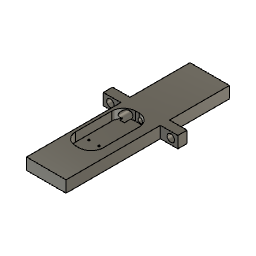
TRAY 3x1.5 v01.1 v3 (Autodesk Fusion 360 design; units mm, degrees)
Autodesk Fusion 360 part; units mm, degrees
sketch "Sketch1" plane through (0, 0, 0) normal (0, 0, 1) x (1, 0, 0)
  line L0 (0, 0) -> (43, 0)
  line L1 (43, 0) -> (43, 177.8)
  line L2 (43, 177.8) -> (0, 177.8)
  line L3 (0, 177.8) -> (0, 0)
  line L4 (0, 112.616) -> (-19.05, 112.616)
  line L5 (-19.05, 112.616) -> (-19.05, 102.616)
  line L6 (-19.05, 102.616) -> (0, 102.616)
  line L7 (0, 102.616) -> (0, 112.616)
  line L8 (43, 112.616) -> (62.05, 112.616)
  line L9 (62.05, 112.616) -> (62.05, 102.616)
  line L10 (62.05, 102.616) -> (43, 102.616)
  line L11 (43, 102.616) -> (43, 112.616)
  dimension "d1" = 177.8
  dimension "d2" = 43
  dimension "d5" = 75.184
  dimension "d6" = 75.184
  dimension "d7" = 10
  dimension "d8" = 10
  dimension "d9" = 19.05
  dimension "d10" = 19.05
  constraint horizontal L0
  constraint vertical L1
  constraint horizontal L2
  constraint vertical L3
  constraint coincident L0.start L3.end
  constraint horizontal L4
  constraint vertical L5
  constraint horizontal L6
  constraint vertical L7
  constraint coincident L3 L4.start
  constraint horizontal L8
  constraint vertical L9
  constraint horizontal L10
  constraint vertical L11
  constraint coincident L1 L8.start
  measures "d1" distance of L0.start L2.end
  measures "d2" distance of L1.end L2.end
  measures "d5" distance of L2.end L6
  measures "d6" distance of L2 L10
  measures "d7" distance of L4.end L5.end
  measures "d8" distance of L8.end L9.end
  measures "d9" distance of L4.start L4.end
  measures "d10" distance of L8.start L8.end
extrude "Extrude1" add sketch "Sketch1" along normal blind 12.6
sketch "Sketch2" plane through (0, 0, 12.6) normal (0, 0, 1) x (-1, 0, 0)
  line L0 (-43, -112.616) -> (-43, -177.8)
  line L1 (-43, -177.8) -> (0, -177.8)
  line L2 (0, -177.8) -> (0, -112.616)
  line L3 (0, -112.616) -> (19.05, -112.616)
  line L4 (19.05, -112.616) -> (19.05, -102.616)
  line L5 (19.05, -102.616) -> (0, -102.616)
  line L6 (0, -102.616) -> (0, 0)
  line L7 (0, 0) -> (-43, 0)
  line L8 (-43, 0) -> (-43, -102.616)
  line L9 (-43, -102.616) -> (-62.05, -102.616)
  line L10 (-62.05, -102.616) -> (-62.05, -112.616)
  line L11 (-62.05, -112.616) -> (-43, -112.616)
  line L12 (-3, -102.616) -> (-33, -102.616)
  line L13 (-33, -102.616) -> (-33, -37.316)
  line L14 (-33, -37.316) -> (-3, -37.316)
  line L15 (-3, -37.316) -> (-3, -102.616)
  dimension "d11" = 3
  dimension "d20" = 10
  dimension "d66" = 30
  dimension "d68" = 65.3
  constraint horizontal L12
  constraint vertical L13
  constraint horizontal L14
  constraint vertical L15
  measures "d11" distance of L6 L15
  measures "d20" distance of L3 L12
  measures "d66" distance of L12.start L12.end
  measures "d68" distance of L12.start L14.end
extrude "Extrude2" cut sketch "Sketch2" against normal blind 9.6 contours L12 L13 L14 L15
sketch "Sketch4" plane through (0, 0, 12.6) normal (0, 0, 1) x (-1, 0, 0)
  line L0 (-33, -102.616) -> (-33, -37.316)
  line L1 (-33, -37.316) -> (-3, -37.316)
  line L2 (-3, -37.316) -> (-3, -102.616)
  line L3 (-3, -102.616) -> (-33, -102.616)
  line L4 (-43, -112.616) -> (-43, -177.8)
  line L5 (-43, -177.8) -> (0, -177.8)
  line L6 (0, -177.8) -> (0, -112.616)
  line L7 (0, -112.616) -> (19.05, -112.616)
  line L8 (19.05, -112.616) -> (19.05, -102.616)
  line L9 (19.05, -102.616) -> (0, -102.616)
  line L10 (0, -102.616) -> (0, 0)
  line L11 (0, 0) -> (-43, 0)
  line L12 (-43, 0) -> (-43, -102.616)
  line L13 (-43, -102.616) -> (-62.05, -102.616)
  line L14 (-62.05, -102.616) -> (-62.05, -112.616)
  line L15 (-62.05, -112.616) -> (-43, -112.616)
  line L16 (0, -102.616) -> (-43, -102.616)
  line L17 (-43, -102.616) -> (-43, 0)
  line L18 (-43, 0) -> (0, 0)
  line L19 (0, 0) -> (0, -102.616)
  constraint horizontal L16
  constraint vertical L17
  constraint horizontal L18
  constraint vertical L19
  constraint coincident L11.end L12.start
  constraint coincident L10 L9.end
  constraint coincident L12.end L13.start
sketch "Sketch5" plane through (0, 177.8, 0) normal (0, 1, 0) x (-1, 0, 0)
  line L0 (-43, 0) -> (0, 0)
  line L1 (0, 0) -> (0, 12.6)
  line L2 (0, 12.6) -> (-43, 12.6)
  line L3 (-43, 12.6) -> (-43, 0)
  circle A0 centre (-21.5, 6.3) radius 2.7
  dimension "d21" = 5.4
  dimension "d22" = 6.3
  measures "d21" diameter of A0
  measures "d22" distance of L0 A0.centre
sketch "Sketch6" plane through (0, 0, 3) normal (0, 0, 1) x (-1, 0, 0)
  line L0 (-3, -37.316) -> (-33, -37.316)
  line L1 (-33, -37.316) -> (-33, -102.616)
  line L2 (-33, -102.616) -> (-3, -102.616)
  line L3 (-3, -102.616) -> (-3, -37.316)
  line L4 (-20.5, -102.616) -> (-22.5, -102.616)
  line L5 (-22.5, -102.616) -> (-22.5, -37.316)
  line L6 (-22.5, -37.316) -> (-20.5, -37.316)
  line L7 (-20.5, -37.316) -> (-20.5, -102.616)
  line L8 (-43, -102.616) -> (-43, 0)
  line L9 (-3, -52.308) -> (-33, -52.308)
  line L10 (-33, -52.308) -> (-33, -50.308)
  line L11 (-33, -50.308) -> (-3, -50.308)
  line L12 (-3, -50.308) -> (-3, -52.308)
  line L13 (-43, 0) -> (0, 0)
  dimension "d25" = 2
  dimension "d26" = 20.5
  dimension "d27" = 2
  dimension "d28" = 50.308
  constraint horizontal L4
  constraint vertical L5
  constraint horizontal L6
  constraint vertical L7
  constraint coincident L0 L5.end
  constraint coincident L2 L4.start
  constraint horizontal L9
  constraint vertical L10
  constraint horizontal L11
  constraint vertical L12
  constraint coincident L1 L10.end
  constraint coincident L3 L9.start
  measures "d25" distance of L5 L7
  measures "d26" distance of L5 L8
  measures "d27" distance of L9 L11
  measures "d28" distance of L11 L13
sketch "Sketch7" plane through (0, 112.616, 0) normal (0, 1, 0) x (-1, 0, 0)
  line L0 (0, 0) -> (19.05, 0)
  line L1 (19.05, 0) -> (19.05, 12.6)
  line L2 (19.05, 12.6) -> (0, 12.6)
  line L3 (0, 12.6) -> (0, 0)
  circle A0 centre (11.356, 6.3008) radius 4.05
  circle A1 centre (-54.3538, 6.3008) radius 4.05
  line L4 (-43, 0) -> (-43, 12.6)
  line L5 (-62.05, 12.6) -> (-43, 12.6)
  dimension "d31" = 8.1
  dimension "d32" = 8.1
  dimension "d33" = 65.7098
  dimension "d34" = 11.3538
  dimension "d37" = 6.2992
  dimension "d38" = 6.2992
  measures "d31" diameter of A1
  measures "d32" diameter of A0
  measures "d33" distance of A0.centre A1.centre
  measures "d34" distance of A1.centre L4
  measures "d37" distance of L2 A0.centre
  measures "d38" distance of A1.centre L5
extrude "Extrude6" cut sketch "Sketch7" against normal blind 12.7 contours A0 | A1
sketch "Sketch8" plane through (0, 0, 3) normal (0, 0, 1) x (-1, 0, 0)
  line L0 (-3, -102.616) -> (-3, -37.316)
  line L1 (-3, -37.316) -> (-33, -37.316)
  circle A0 centre (-8, -59.652) radius 1
  circle A1 centre (-19.176, -59.652) radius 1
  circle A2 centre (-19.176, -42.964) radius 1
  circle A3 centre (-8, -42.964) radius 1
  line L2 (-2, -52.308) -> (-20.5, -52.308)
  line L3 (-33, -37.316) -> (-33, -102.616)
  line L4 (-33, -102.616) -> (-3, -102.616)
  dimension "d39" = 2
  dimension "d41" = 2
  dimension "d44" = 11.176
  dimension "d45" = 2
  dimension "d46" = 16.688
  dimension "d48" = 2
  dimension "d49" = 16.688
  dimension "d50" = 11.176
  dimension "d64" = 7.344
  dimension "d65" = 7.344
  dimension "d69" = 5
  measures "d39" diameter of A0
  measures "d41" diameter of A1
  measures "d44" distance of A0.centre A1.centre
  measures "d45" diameter of A2
  measures "d46" vertical distance of A1.centre A2.centre
  measures "d48" diameter of A3
  measures "d49" vertical distance of A0.centre A3.centre
  measures "d50" distance of A2.centre A3.centre
  measures "d64" distance of A0.centre L2
  measures "d65" distance of A1.centre L2
  measures "d69" distance of L0 A0.centre
extrude "Extrude7" cut sketch "Sketch8" against normal blind 4 contours A0 | A1 | A2 | A3
sketch "Sketch9" plane through (0, 177.8, 0) normal (0, 1, 0) x (-1, 0, 0)
  line L0 (-43, 0) -> (0, 0)
  line L1 (0, 0) -> (0, 12.6)
  line L2 (0, 12.6) -> (-43, 12.6)
  line L3 (-43, 12.6) -> (-43, 0)
  line L4 (-43, 1.27) -> (0, 1.27)
  line L5 (0, 1.27) -> (0, 0)
  line L6 (0, 0) -> (-43, 0)
  line L7 (-43, 0) -> (-43, 1.27)
  dimension "d53" = 1.27
  constraint horizontal L4
  constraint vertical L5
  constraint horizontal L6
  constraint vertical L7
  constraint coincident L0.end L1.start
  constraint coincident L3 L4.start
  measures "d53" distance of L4 L6
sketch "Sketch10" plane through (0, 0, 0) normal (0, -1, 0) x (1, 0, 0)
  line L0 (0, 12.6) -> (0, 0)
  line L1 (0, 0) -> (43, 0)
  line L2 (43, 0) -> (43, 12.6)
  line L3 (43, 0) -> (0, 0)
  line L4 (0, 0) -> (0, 1.27)
  line L5 (43, 1.27) -> (43, 0)
  line L6 (0, 1.27) -> (43, 1.27)
  line L7 (43, 12.6) -> (0, 12.6)
  dimension "d56" = 1.27
  constraint horizontal L3
  constraint coincident L1.end L2.start
  constraint coincident L0.end L1.start
  constraint coincident L0 L4.end
  constraint coincident L2 L5.start
  constraint perpendicular L5 L6
  measures "d56" distance of L3 L6
thread "Thread1" "ANSI Metric M Profile 2.0 M2x0.4 6H" major diameter 2.074 minor diameter 1.623 pitch 0.4 angle 60 modelled right hand crest width 0.1065 on face at (7.0785, 59.2636, 1) crest through (7.1885, 59.652, 2.9)
thread "Thread2" "ANSI Metric M Profile 2.0 M2x0.4 6H" major diameter 2.074 minor diameter 1.623 pitch 0.4 angle 60 modelled right hand crest width 0.1065 on face at (20.1157, 59.994, 1) crest through (18.3645, 59.652, 2.9)
thread "Thread3" "ANSI Metric M Profile 2.0 M2x0.4 6H" major diameter 2.074 minor diameter 1.623 pitch 0.4 angle 60 modelled right hand crest width 0.1065 on face at (20.1157, 43.306, 1) crest through (18.3645, 42.964, 2.9)
thread "Thread4" "ANSI Metric M Profile 2.0 M2x0.4 6H" major diameter 2.074 minor diameter 1.623 pitch 0.4 angle 60 modelled right hand crest width 0.1065 on face at (7.0785, 42.5756, 1) crest through (7.1885, 42.964, 2.9)
sketch "Sketch11" plane through (0, 177.8, 0) normal (0, 1, 0) x (-1, 0, 0)
  line L0 (0, 0) -> (0, 12.6)
  line L1 (0, 12.6) -> (-43, 12.6)
  line L2 (-43, 12.6) -> (-43, 0)
  circle A0 centre (-8.8291, 6.758) radius 4.5
  line L3 (-43, 0) -> (0, 0)
  dimension "d59" = 9
  dimension "d60" = 5.842
  measures "d59" diameter of A0
  measures "d60" distance of L1 A0.centre
fillet "Fillet1" radius 13 4 edges at (3, 37.316, 7.8) (33, 37.316, 7.8) (33, 102.616, 7.8) (3, 102.616, 7.8)
extrude "Extrude11" cut sketch "Sketch5" against normal blind 76.2 contours A0
extrude "Extrude12" cut sketch "Sketch11" against normal blind 82.55 contours A0
